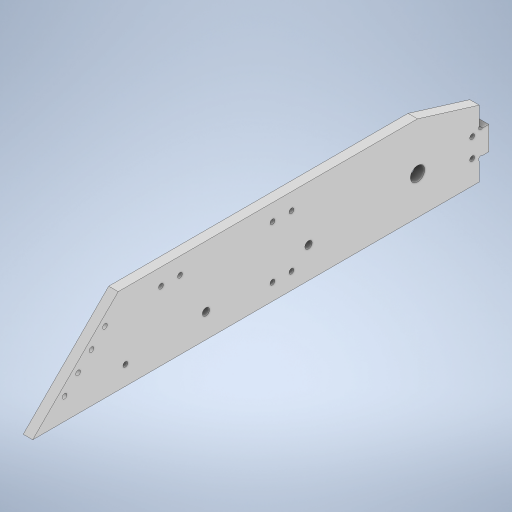
# Autodesk Inventor part: Side Wall_outer
Saved by Autodesk Inventor 2023 (Build 270158000, 158)
## iProperties
Created: 2022-12-26
Part Number: Side Wall_outer
Material: Generic
Document SubType Name: Modeling
Designer: justi
Density: 1 g/cm^3
Appearance: Default
Mass: 769.938 g
Surface Area: 1403.11 cm^2
Volume: 769.938 cm^3
Author: justi
Autodesk Inventor part; units mm, degrees
ref_plane "YZ Plane" through (0, 0, 0) normal (1, 0, 0) x (0, 1, 0)
ref_plane "XZ Plane" through (0, 0, 0) normal (0, 1, 0) x (-1, 0, 0)
ref_plane "XY Plane" through (0, 0, 0) normal (0, 0, 1) x (1, 0, 0)
sketch "Sketch1" plane through (0, 0, 0) normal (1, 0, 0) x (0, 1, 0)
  line L0 (0, 0) -> (101.6, 0)
  line L1 (101.6, 0) -> (101.6, -508)
  line L2 (101.6, -508) -> (0, -508)
  line L3 (0, -508) -> (0, 0)
  line L4 (0, 0) -> (0, 101.6)
  line L5 (0, 101.6) -> (101.6, 0)
  line L6 (101.6, -508) -> (114.3, -508)
  line L7 (114.3, -508) -> (114.3, -12.7)
  line L8 (114.3, -12.7) -> (101.6, -12.7)
  line L9 (101.6, -12.7) -> (101.6, -508)
  line L10 (114.3, -12.7) -> (101.6, 0)
  line L11 (0, -508) -> (28.575, -508)
  line L12 (28.575, -508) -> (28.575, -495.3)
  line L13 (28.575, -495.3) -> (0, -495.3)
  line L14 (0, -495.3) -> (0, -508)
  line L15 (60.325, -508) -> (114.3, -508)
  line L16 (114.3, -508) -> (114.3, -495.3)
  line L17 (114.3, -495.3) -> (60.325, -495.3)
  line L18 (60.325, -495.3) -> (60.325, -508)
  circle A0 centre (50.8, -412.75) radius 9.525
  line L19 (50.8, -412.75) -> (127.2366, -412.75)
  line L20 (114.3, -412.75) -> (88.9, -495.3)
  point P0 (0, -495.3)
  dimension "d0" = 508
  dimension "d1" = 101.6
  dimension "d2" = 101.6
  dimension "d3" = 12.7
  dimension "d4" = 495.3
  dimension "d5" = 28.575
  dimension "d6" = 12.7
  dimension "d7" = 31.75
  dimension "d8" = 19.05
  dimension "d9" = 95.25
  dimension "d10" = 50.8
  dimension "d11" = 28.575
  dimension "d14" = 12.7
  constraints: 42 end point, 8 parallel, 5 perpendicular, 5 point on line, 4 horizontal, 1 centre point, 1 vertical
  measures "d0" distance of L0.end L1.end
  measures "d1" distance of L1.end L2.end
  measures "d2" distance of L0.start L4.end
  measures "d3" distance of L8.end L7.end
  measures "d4" distance of L6.end L7.end
  measures "d5" distance of L13.end L12.end
  measures "d6" distance of L11.end L12.end
  measures "d7" distance between parallel lines of L12 L18
  measures "d8" diameter of A0
  measures "d9" distance from line of L2 L19.start
  measures "d10" distance from line of L3 L19.start
  measures "d11" distance from line of L18 L20.end
  measures "d14" distance of L17.end L15.start
extrude "Extrusion1" add sketch "Sketch1" along normal blind 12.7 contours L4 L5 L0 | L0 L1 L20 L17 L18 L2 L12 L13 L3 | L10 L8 L1 | L8 L7 L19 L1 | L19 L20 L1
sketch "Sketch2" plane through (12.7, 0, 0) normal (1, 0, 0) x (0, 0, -1)
  line L0 (508, 60.325) -> (495.3, 60.325) projected
  line L1 (495.3, 60.325) -> (497.5451, 62.5701)
  line L2 (495.3, 0) -> (495.3, 28.575) projected
  line L3 (495.3, 28.575) -> (497.5451, 26.3299)
  line L4 (495.3, 28.575) -> (508, 28.575) projected
  circle A0 centre (497.5451, 62.5701) radius 3.175
  circle A1 centre (497.5451, 26.3299) radius 3.175
  point P0 (0, 0)
  dimension "d15" = 3.175
  dimension "d16" = 45
  dimension "d17" = 3.175
  dimension "d18" = 45
  dimension "d19" = 6.35
  dimension "d20" = 6.35
  constraints: 4 end point, 2 centre point, 1 point on line
  measures "d15" distance of L0.end L1.end
  measures "d16" angle of L0 L1
  measures "d17" distance of L2.end L3.end
  measures "d18" angle of L4 L3
  measures "d19" diameter of A0
  measures "d20" diameter of A1
extrude "Extrusion2" cut sketch "Sketch2" against normal blind 12.7
sketch "Sketch3" plane through (12.7, 0, 0) normal (1, 0, 0) x (0, 0, -1)
  circle A0 centre (485.775, 57.15) radius 3.175
  line L0 (495.3, 64.8151) -> (495.3, 88.9) projected
  line L1 (508, 28.575) -> (508, 60.325) projected
  circle A1 centre (485.775, 31.75) radius 3.175
  line L2 (495.3, 0) -> (495.3, 24.0849) projected
  line L3 (12.7, 114.3) -> (-101.6, 0) projected
  line L4 (-83.6395, 17.9605) -> (-29.758, 71.842)
  line L5 (-29.758, 71.842) -> (-16.2876, 58.3717)
  line L6 (-16.2876, 58.3717) -> (-70.1691, 4.4901)
  line L7 (-70.1691, 4.4901) -> (-83.6395, 17.9605)
  circle A2 centre (-58.9438, 29.1858) radius 3.175
  circle A3 centre (-40.9833, 47.1463) radius 3.175
  point P0 (0, 0)
  point P1 (508, 44.45)
  point P2 (508, 44.45)
  dimension "d23" = 6.35
  dimension "d25" = 9.525
  dimension "d27" = 12.7
  dimension "d28" = 6.35
  dimension "d29" = 9.525
  dimension "d30" = 12.7
  dimension "d31" = 19.05
  dimension "d32" = 76.2
  dimension "d33" = 25.4
  dimension "d34" = 6.35
  dimension "d35" = 6.35
  dimension "d36" = 9.525
  dimension "d37" = 9.525
  dimension "d38" = 25.4
  dimension "d39" = 25.4
  constraints: 8 end point, 4 centre point, 2 midpoint, 2 parallel, 2 point on line, 1 perpendicular
  measures "d23" diameter of A0
  measures "d25" distance from line of L0 A0.centre
  measures "d27" vertical distance of point (508, 44.45) A0.centre
  measures "d28" diameter of A1
  measures "d29" distance from line of L2 A1.centre
  measures "d30" vertical distance of point (508, 44.45) A1.centre
  measures "d31" distance of L4.end L5.end
  measures "d32" distance of L5.end L6.end
  measures "d33" distance from line of L3.end L7
  measures "d34" diameter of A2
  measures "d35" diameter of A3
  measures "d36" distance from line of L3 A2.centre
  measures "d37" distance from line of L4 A3.centre
  measures "d38" distance from line of L7 A2.centre
  measures "d39" distance of A3.centre A2.centre
extrude "Extrusion3" cut sketch "Sketch3" against normal blind 12.7 contours A0 | A1 | A2 | A3
sketch "Sketch4" plane through (12.7, 0, 0) normal (1, 0, 0) x (0, 0, -1)
  circle A0 centre (218.821, 92.075) radius 3.175
  line L0 (-101.6, 0) -> (495.3, 0) projected
  circle A1 centre (244.221, 92.075) radius 3.175
  point P0 (0, 0)
  dimension "d42" = 6.35
  dimension "d43" = 92.075
  dimension "d44" = 6.35
  dimension "d45" = 92.075
  dimension "d46" = 218.821
  dimension "d47" = 244.221
  constraints: 2 centre point
  measures "d42" diameter of A0
  measures "d43" distance from line of L0 A0.centre
  measures "d44" diameter of A1
  measures "d45" distance from line of L0 A1.centre
  measures "d46" horizontal distance of point (0, 0) A0.centre
  measures "d47" horizontal distance of point (0, 0) A1.centre
extrude "Extrusion4" cut sketch "Sketch4" against normal blind 12.7
sketch "Sketch6" plane through (12.7, 0, 0) normal (1, 0, 0) x (0, 0, -1)
  circle A0 centre (218.821, 22.225) radius 3.175
  circle A1 centre (244.221, 22.225) radius 3.175
  line L0 (-101.6, 0) -> (495.3, 0) projected
  point P0 (0, 0)
  dimension "d59" = 6.35
  dimension "d60" = 6.35
  dimension "d61" = 218.821
  dimension "d62" = 22.225
  dimension "d63" = 22.225
  dimension "d64" = 25.4
  constraints: 2 centre point
  measures "d59" diameter of A0
  measures "d60" diameter of A1
  measures "d61" horizontal distance of point (0, 0) A0.centre
  measures "d62" distance from line of L0 A0.centre
  measures "d63" distance from line of L0 A1.centre
  measures "d64" distance of A0.centre A1.centre
extrude "Extrusion6" cut sketch "Sketch6" against normal blind 12.7
sketch "Sketch7" plane through (12.7, 0, 0) normal (1, 0, 0) x (0, 0, -1)
  circle A0 centre (69.85, 92.075) radius 3.175
  circle A1 centre (95.25, 92.075) radius 3.175
  line L0 (412.75, 114.3) -> (12.7, 114.3) projected
  point P0 (0, 0)
  dimension "d67" = 6.35
  dimension "d68" = 6.35
  dimension "d69" = 69.85
  dimension "d70" = 22.225
  dimension "d71" = 22.225
  dimension "d72" = 25.4
  constraints: 2 centre point
  measures "d67" diameter of A0
  measures "d68" diameter of A1
  measures "d69" horizontal distance of point (0, 0) A0.centre
  measures "d70" distance from line of L0 A0.centre
  measures "d71" distance from line of L0 A1.centre
  measures "d72" distance of A0.centre A1.centre
extrude "Extrusion7" cut sketch "Sketch7" against normal blind 12.7
sketch "Sketch10" plane through (12.7, 0, 0) normal (1, 0, 0) x (0, 0, -1)
  circle A0 centre (22.225, 25.4) radius 3.175
  line L0 (-101.6, 0) -> (495.3, 0) projected
  circle A1 centre (412.75, 50.8) radius 9.525 projected
  circle A2 centre (412.75, 50.8) radius 76.2
  circle A3 centre (22.225, 25.4) radius 38.1
  line L1 (22.225, 25.4) -> (412.75, 50.8)
  circle A4 centre (129.9474, 32.4063) radius 4.7625
  circle A5 centre (267.0079, 41.3208) radius 4.7625
  point P0 (0, 0)
  dimension "d82" = 6.35
  dimension "d83" = 25.4
  dimension "d84" = 22.225
  dimension "d85" = 152.4
  dimension "d86" = 76.2
  dimension "d87" = 9.525
  dimension "d88" = 107.95
  dimension "d89" = 9.525
  dimension "d90" = 146.05
  constraints: 5 centre point, 2 coincident, 2 end point, 2 point on line
  measures "d82" diameter of A0
  measures "d83" distance from line of L0 A0.centre
  measures "d84" horizontal distance of point (0, 0) A0.centre
  measures "d85" diameter of A2
  measures "d86" diameter of A3
  measures "d87" diameter of A4
  measures "d88" distance of A0.centre A4.centre
  measures "d89" diameter of A5
  measures "d90" distance of L1.end A5.centre
extrude "Extrusion8" cut sketch "Sketch10" against normal blind 12.7 contours A0 | A4 L1 | L1 A4 | A5 L1 | L1 A5
sketch "Sketch15" plane through (12.7, 0, 0) normal (1, 0, 0) x (0, 0, -1)
  circle A0 centre (-23.0228, 65.1069) radius 3.175
  line L0 (12.7, 114.3) -> (-101.6, 0) projected
  circle A1 centre (-40.9833, 47.1463) radius 3.175 projected
  circle A2 centre (-5.0622, 83.0674) radius 3.175
  line L1 (-74.6592, 26.9408) -> (-2.8172, 98.7828)
  line L2 (-2.8172, 98.7828) -> (10.6532, 85.3124)
  line L3 (10.6532, 85.3124) -> (-61.1888, 13.4704)
  line L4 (-61.1888, 13.4704) -> (-74.6592, 26.9408)
  circle A3 centre (-58.9438, 29.1858) radius 3.175 projected
  point P0 (0, 0)
  dimension "d103" = 6.35
  dimension "d104" = 9.525
  dimension "d105" = 25.4
  dimension "d106" = 6.35
  dimension "d107" = 9.525
  dimension "d108" = 25.4
  dimension "d109" = 19.05
  dimension "d110" = 12.7
  dimension "d111" = 101.6
  constraints: 8 end point, 2 centre point, 2 parallel, 2 point on line, 1 perpendicular
  measures "d103" diameter of A0
  measures "d104" distance from line of L0 A0.centre
  measures "d105" distance of A1.centre A0.centre
  measures "d106" diameter of A2
  measures "d107" distance from line of L0 A2.centre
  measures "d108" distance of A0.centre A2.centre
  measures "d109" distance of L1.end L2.end
  measures "d110" distance from line of A3.centre L4
  measures "d111" distance of L2.end L3.end
extrude "Extrusion11" cut sketch "Sketch15" against normal blind 12.7 contours A0 | A2
body "Solid1"
